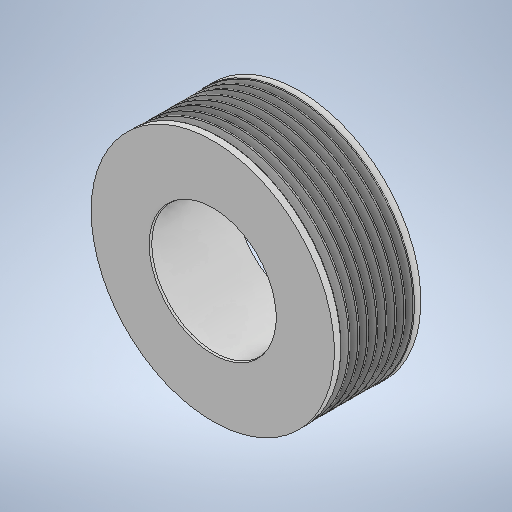
# Autodesk Inventor part: 29-10-202
Saved by Autodesk Inventor 2025.2 (Build 292293000, 293)
## iProperties
Created: 2024-11-27
Part Number: 29-10-202
Material: Generic
Document SubType Name: Modeling
Designer: Zvonko.Gabric
Density: 1 g/cm^3
Appearance: Default
Description: Polly-V PJ8 22mm
Author: Zvonko.Gabric
Autodesk Inventor part; units mm, degrees
ref_plane "YZ Plane" through (0, 0, 0) normal (1, 0, 0) x (0, 1, 0)
ref_plane "XZ Plane" through (0, 0, 0) normal (0, 1, 0) x (-1, 0, 0)
ref_plane "XY Plane" through (0, 0, 0) normal (0, 0, 1) x (1, 0, 0)
sketch "Sketch1" plane through (0, 0, 0) normal (0, 1, 0) x (-1, 0, 0)
  line L0 (-6.9498, 24.8127) -> (-6.8158, 25.3127)
  line L1 (-6.9498, 3.4467) -> (-6.9498, 24.8127)
  line L2 (-6.4498, 3.3127) -> (-6.9498, 3.4467)
  line L3 (5.9466, 22.8034) -> (5.9466, 22.202)
  arc A0 (5.9466, 8.7634) -> (5.9466, 8.162) centre (6.056, 8.4627) ccw
  arc A1 (5.9466, 11.1034) -> (5.9466, 10.502) centre (6.056, 10.8027) ccw
  arc A2 (5.9466, 13.4434) -> (5.9466, 12.842) centre (6.056, 13.1427) ccw
  arc A3 (5.9466, 15.7834) -> (5.9466, 15.182) centre (6.056, 15.4827) ccw
  arc A4 (5.9466, 18.1234) -> (5.9466, 17.522) centre (6.056, 17.8227) ccw
  arc A5 (5.9466, 20.4634) -> (5.9466, 19.862) centre (6.056, 20.1627) ccw
  line L4 (-6.8158, 25.3127) -> (7.9502, 25.3127)
  line L5 (5.9466, 22.202) -> (7.8186, 21.5206)
  arc A6 (7.8186, 21.1448) -> (7.8186, 21.5206) centre (7.7502, 21.3327) ccw
  line L6 (7.8186, 21.1448) -> (5.9466, 20.4634)
  line L7 (5.9466, 19.862) -> (7.8186, 19.1806)
  arc A7 (7.8186, 18.8048) -> (7.8186, 19.1806) centre (7.7502, 18.9927) ccw
  line L8 (7.8186, 18.8048) -> (5.9466, 18.1234)
  line L9 (5.9466, 17.522) -> (7.8186, 16.8406)
  arc A8 (7.8186, 16.4648) -> (7.8186, 16.8406) centre (7.7502, 16.6527) ccw
  line L10 (7.8186, 16.4648) -> (5.9466, 15.7834)
  line L11 (7.9502, 3.3127) -> (-6.4498, 3.3127)
  line L12 (5.9466, 15.182) -> (7.8186, 14.5006)
  line L13 (7.9502, 4.9527) -> (7.9502, 3.3127)
  line L14 (5.9466, 5.822) -> (7.8186, 5.1406)
  line L15 (7.8186, 9.4448) -> (5.9466, 8.7634)
  line L16 (7.8186, 7.1048) -> (5.9466, 6.4234)
  line L17 (5.9466, 8.162) -> (7.8186, 7.4806)
  arc A9 (7.8186, 7.1048) -> (7.8186, 7.4806) centre (7.7502, 7.2927) ccw
  arc A10 (7.9502, 4.9527) -> (7.8186, 5.1406) centre (7.7502, 4.9527) ccw
  arc A11 (5.9466, 22.8034) -> (5.9466, 22.202) centre (6.056, 22.5027) ccw
  line L18 (7.8186, 23.4848) -> (5.9466, 22.8034)
  line L19 (7.9502, 25.3127) -> (7.9502, 23.6727)
  arc A12 (7.8186, 23.4848) -> (7.9502, 23.6727) centre (7.7502, 23.6727) ccw
  arc A13 (5.9466, 6.4234) -> (5.9466, 5.822) centre (6.056, 6.1227) ccw
  line L20 (5.9466, 10.502) -> (7.8186, 9.8206)
  arc A14 (7.8186, 9.4448) -> (7.8186, 9.8206) centre (7.7502, 9.6327) ccw
  line L21 (7.8186, 14.1248) -> (5.9466, 13.4434)
  arc A15 (7.8186, 14.1248) -> (7.8186, 14.5006) centre (7.7502, 14.3127) ccw
  line L22 (7.8186, 11.7848) -> (5.9466, 11.1034)
  arc A16 (7.8186, 11.7848) -> (7.8186, 12.1606) centre (7.7502, 11.9727) ccw
  line L23 (5.9466, 12.842) -> (7.8186, 12.1606)
  line L24 (-6.9498, 14.1297) -> (-22.9498, 14.1297) construction
  line L25 (-22.9498, 26.3581) -> (-22.9498, -3.8355) construction
  point P0 (0, 0)
  point P1 (7.9502, 24.4927)
  point P2 (5.9466, 22.5027)
  dimension "d2" = 16
  dimension "d4" = 22
  dimension "d5" = 14.9
  dimension "d6" = 40
  dimension "d7" = 14.4
  dimension "d8" = 105
  dimension "d9" = 13.0058
  dimension "d10" = 2.34
  dimension "d11" = 2.81
  dimension "d12" = 16.38
  dimension "d13" = 0.5
  dimension "d14" = 0.134
  dimension "d15" = 90
  dimension "d16" = 105
  dimension "d17" = 0.5
  dimension "d18" = 90
  dimension "d19" = 14.7
  dimension "d20" = 13.0058
  dimension "d21" = 13.0058
  dimension "d22" = 13.0058
  dimension "d23" = 1.64
  dimension "d24" = 20
  dimension "d25" = 0.32
  dimension "d26" = 0.2
  dimension "d27" = 0.32
  dimension "d28" = 0.2
  dimension "d29" = 0.32
  dimension "d30" = 0.2
  dimension "d31" = 0.32
  dimension "d32" = 0.2
  dimension "d33" = 0.32
  dimension "d34" = 0.2
  dimension "d35" = 0.32
  dimension "d36" = 0.2
  dimension "d37" = 0.32
  dimension "d38" = 0.2
  dimension "d39" = 0.2
  dimension "d40" = 1.64
  dimension "d41" = 40
  dimension "d42" = 0.32
  dimension "d43" = 1.64
  dimension "d44" = 0.2
  dimension "d45" = 40
  dimension "d46" = 40
  dimension "d47" = 40
  dimension "d48" = 40
  dimension "d49" = 40
  dimension "d50" = 40
  dimension "d51" = 14.7
  dimension "d52" = 2.34
  dimension "d53" = 2.34
  dimension "d54" = 2.34
  dimension "d55" = 2.34
  dimension "d56" = 2.34
  dimension "d57" = 2.34
  dimension "d58" = 2.81
  dimension "d59" = 1.872
  dimension "d60" = 1.872
  dimension "d61" = 1.872
  dimension "d62" = 0.6814
  dimension "d63" = 1.872
  dimension "d64" = 2.34
  dimension "d65" = 1.872
  dimension "d66" = 1.872
  constraints: 52 end point, 34 point on circle, 17 centre point, 3 midpoint, 1 horizontal, 1 vertical
  measures "d2" distance of L24.start L24.end
  measures "d4" distance between parallel lines of L4 L11
  measures "d5" distance from line of point (7.95, 24.493) L1
  measures "d6" angle of L5 L18
  measures "d7" distance of L11.start L2.start
  measures "d8" angle of L4 L0
  measures "d9" distance from line of L1 A13.centre
  measures "d10" distance of A5.centre A11.centre
  measures "d11" distance from line of L4 A11.centre
  measures "d12" vertical distance of point (5.947, 22.503) A13.centre
  measures "d13" vertical distance of L0.start L0.end
  measures "d14" horizontal distance of L0.start L0.end
  measures "d15" angle of L4 L19
  measures "d16" angle of L1 L2
  measures "d17" horizontal distance of L2.start L1.start
  measures "d18" angle of L13 L11
  measures "d19" distance from line of L1 A10.centre
  measures "d20" distance from line of L1 A2.centre
  measures "d21" distance from line of L1 A1.centre
  measures "d22" distance from line of L1 A0.centre
  measures "d23" distance from line of L4 A12.centre
  measures "d24" angle of L18 L4
  measures "d25" radius of A11
  measures "d26" radius of A6
  measures "d27" radius of A5
  measures "d28" radius of A7
  measures "d29" radius of A4
  measures "d30" radius of A8
  measures "d31" radius of A3
  measures "d32" radius of A15
  measures "d33" radius of A2
  measures "d34" radius of A16
  measures "d35" radius of A1
  measures "d36" radius of A14
  measures "d37" radius of A0
  measures "d38" radius of A9
  measures "d39" radius of A12
  measures "d40" distance of L4.end L19.end
  measures "d41" angle of L14 L16
  measures "d42" radius of A13
  measures "d43" distance of L13.start L11.start
  measures "d44" radius of A10
  measures "d45" angle of L7 L6
  measures "d46" angle of L9 L8
  measures "d47" angle of L12 L10
  measures "d48" angle of L23 L21
  measures "d49" angle of L20 L22
  measures "d50" angle of L17 L15
  measures "d51" distance from line of L1 A9.centre
  measures "d52" distance of A4.centre A5.centre
  measures "d53" distance of A3.centre A4.centre
  measures "d54" distance of A2.centre A3.centre
  measures "d55" distance of A1.centre A2.centre
  measures "d56" distance of A0.centre A1.centre
  measures "d57" distance of A13.centre A0.centre
  measures "d58" distance from line of L11 A13.centre
  measures "d59" horizontal distance of L18.start L3.start
  measures "d60" horizontal distance of L3.end L5.end
  measures "d61" horizontal distance of L6.start L6.end
  measures "d62" vertical distance of L7.start L7.end
  measures "d63" horizontal distance of L7.start L7.end
  measures "d64" distance of A14.centre A9.centre
  measures "d65" horizontal distance of L20.start L20.end
  measures "d66" horizontal distance of L22.start L22.end
revolve "Revolution1" add sketch "Sketch1" angle 360 about axis through (22.9498, 0, 26.3581) along (0, 0, -1) contours L0 L4 L19 A12 L18 A11 L5 A6 L6 A5 L7 A7 L8 A4 L9 A8 L10 A3 L12 A15 L21 A2 L23 A16 L22 A1 L20 A14 L15 A0 L17 A9 L16 A13 L14 A10 L13 L11 L2 L1
body "Solid1"
